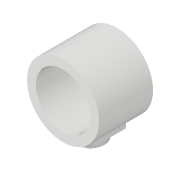
# Autodesk Inventor part: Part4
Saved by Autodesk Inventor 2017 (Build 210142000, 142)
## iProperties
Created: 2017-05-11
Part Number: Part4
Material: ABS Plastic
Document SubType Name: Modeling
Designer: zallen
Density: 1.06 g/cm^3
Appearance: Smooth - White
Mass: 297.541 g
Surface Area: 505.311 cm^2
Volume: 280.699 cm^3
Author: zallen
Autodesk Inventor part; units mm, degrees
ref_plane "YZ Plane" through (0, 0, 0) normal (1, 0, 0) x (0, 1, 0)
ref_plane "XZ Plane" through (0, 0, 0) normal (0, 1, 0) x (-1, 0, 0)
ref_plane "XY Plane" through (0, 0, 0) normal (0, 0, 1) x (1, 0, 0)
sketch "Sketch1" plane through (0, 0, 0) normal (0, 0, 1) x (1, 0, 0)
  circle A0 centre (0, 0) radius 50
  dimension "d0" = 100
  constraints: 1 centre point, 1 coincident
  measures "d0" diameter of A0
extrude "Extrusion1" add sketch "Sketch1" along normal mid plane 75
sketch "Sketch2" plane through (0, 0, 37.5) normal (0, 0, 1) x (1, 0, 0)
  circle A0 centre (0, 0) radius 37.5
  dimension "d3" = 75
  constraints: 1 centre point, 1 coincident
  measures "d3" diameter of A0
extrude "Extrusion2" cut sketch "Sketch2" against normal through all
sketch "Sketch4" plane through (0, 0, 0) normal (0, 0, 1) x (1, 0, 0)
  line L0 (25, -43.3013) -> (25, -52)
  line L1 (25, -52) -> (-25, -52)
  line L2 (-25, -52) -> (-25, -43.3013)
  arc A0 (-25, -43.3013) -> (25, -43.3013) centre (0, 0) ccw
  circle A1 centre (0, 0) radius 50 projected
  line L3 (0, 0) -> (0, -66.2618) construction
  dimension "d22" = 50
  dimension "d24" = 90
  dimension "d25" = 50
  dimension "d26" = 52
  constraints: 8 end point, 4 point on circle, 2 perpendicular, 2 vertical, 1 centre point, 1 other
  measures "d22" distance of L0.end L1.end
  measures "d24" angle of L1 L2
  measures "d25" radius of A0
  measures "d26" distance from line of point (0, 0) L1
extrude "Extrusion3" add sketch "Sketch4" along normal mid plane 50 contours L0 L1 L2 A0
sketch "Sketch6" plane through (-25, -52, 25) normal (0, -1, 0) x (1, 0, 0)
  circle A0 centre (25, -25) radius 20
  dimension "d27" = 40
  constraints: 1 centre point, 1 coincident
  measures "d27" diameter of A0
extrude "Extrusion5" add sketch "Sketch6" along normal blind 10
body "Solid1"
